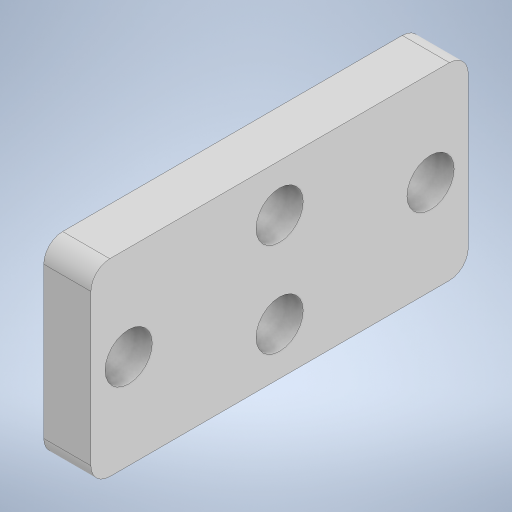
# Autodesk Inventor part: perno
Saved by Autodesk Inventor 2023 (Build 270158000, 158)
## iProperties
Created: 2023-08-01
Part Number: perno
Material: Generico
Document SubType Name: Modeling
Designer: Admin
Density: 1 g/cm^3
Appearance: Default
Author: Admin
Autodesk Inventor part; units mm, degrees
ref_plane "YZ Plane" through (0, 0, 0) normal (1, 0, 0) x (0, 1, 0)
ref_plane "XZ Plane" through (0, 0, 0) normal (0, 1, 0) x (-1, 0, 0)
ref_plane "XY Plane" through (0, 0, 0) normal (0, 0, 1) x (1, 0, 0)
sketch "Schizzo1" plane through (0, 0, 0) normal (1, 0, 0) x (0, 1, 0)
  line L0 (10, 20) -> (-10, 20)
  line L1 (-10, 20) -> (-10, -20)
  line L2 (-10, -20) -> (10, -20)
  line L3 (10, -20) -> (10, 20)
  line L4 (0, 0) -> (10, 0) construction
  line L5 (0, 0) -> (0, -19.4896) construction
  circle A0 centre (0, 16) radius 2.5
  circle A1 centre (0, -16) radius 2.5
  circle A2 centre (5, 0) radius 2.5
  circle A3 centre (-5, 0) radius 2.5
  dimension "d0" = 40
  dimension "d1" = 20
  dimension "d2" = 4
  dimension "d3" = 5
  dimension "d8" = 5
  dimension "d9" = 5
  dimension "d10" = 5
  dimension "d11" = 10
  constraints: 12 end point, 4 centre point, 2 horizontal, 2 parallel, 1 midpoint, 1 perpendicular, 1 point on line, 1 symmetric about line, 1 vertical, 3 other
  measures "d0" distance of L2.end L0.start
  measures "d1" distance of L0.start L0.end
  measures "d2" distance from line of L0 A0.centre
  measures "d3" diameter of A0
  measures "d8" diameter of A2
  measures "d9" diameter of A3
  measures "d10" distance from line of A2.centre L3
  measures "d11" distance of A3.centre A2.centre
extrude "Estrusione1" add sketch "Schizzo1" along normal mid plane 5 contours L3 L2 L1 L0 | A2 | A3
fillet "Raccordo1" radius 2 4 edges at (0, 10, 20) (0, -10, 20) (0, 10, -20) (0, -10, -20)
extrude "Estrusione2" cut sketch "Schizzo1" along normal mid plane 5 contours A2 | A3
